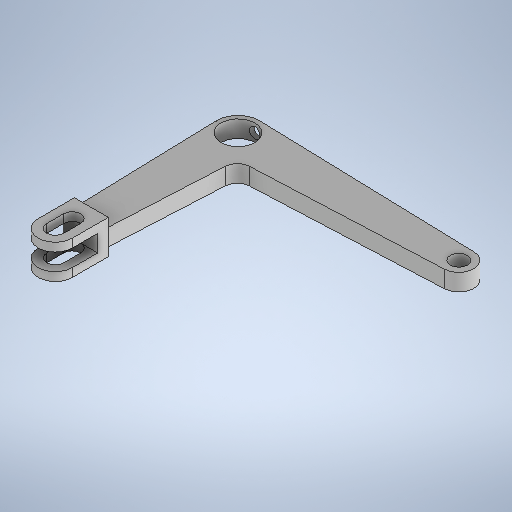
# Autodesk Inventor part: 10
Saved by Autodesk Inventor 2025.1 (Build 291241000, 241)
## iProperties
Created: 2024-09-12
Part Number: 10
Material: Generisch
Document SubType Name: Modeling
Designer: ffogue
Density: 1 g/cm^3
Appearance: Vorgabe
Author: ffogue
Autodesk Inventor part; units mm, degrees
ref_plane "YZ Plane" through (0, 0, 0) normal (1, 0, 0) x (0, 1, 0)
ref_plane "XZ Plane" through (0, 0, 0) normal (0, 1, 0) x (-1, 0, 0)
sketch "Sketch2" plane through (0, 0, 0) normal (0, 0, 1) x (1, 0, 0)
  line L0 (-4, 0) -> (4, 0)
  line L1 (4, 0) -> (4, -12.5)
  line L2 (4, -12.5) -> (-4, -12.5)
  line L3 (-4, -12.5) -> (-4, 0)
  point P0 (0, 0)
  point P1 (0, 0)
  dimension "d8" = 12.5
  dimension "d9" = 8
  constraints: 8 end point, 2 parallel, 1 coincident, 1 horizontal, 1 midpoint, 1 perpendicular
  measures "d8" distance between parallel lines of L2 L0
  measures "d9" distance of L0.start L0.end
extrude "Extrusion1" add sketch "Sketch2" along normal mid plane 8
fillet "Fillet1" radius 4 2 edges at (4, -12.5, 0) (-4, -12.5, 0)
sketch "Sketch4" plane through (0, 0, 4) normal (0, 0, 1) x (1, 0, 0)
  line L0 (0, -8.5) -> (0, -4.5) construction
  line L1 (2, -8.5) -> (2, -4.5)
  line L2 (-2, -4.5) -> (-2, -8.5)
  arc A0 (-2, -8.5) -> (2, -8.5) centre (0, -8.5) ccw
  arc A1 (2, -4.5) -> (-2, -4.5) centre (0, -4.5) ccw
  line L3 (4, 0) -> (-4, 0) projected
  point P0 (0, 0)
  point P1 (0, -6.5)
  point P2 (0, 0)
  dimension "d17" = 4
  dimension "d18" = 2
  constraints: 8 end point, 4 point on circle, 4 tangent, 2 centre point, 2 midpoint, 1 parallel, 1 vertical, 1 vertical alignment
  measures "d17" distance of L0.start L0.end
  measures "d18" radius of A0
extrude "Extrusion3" cut sketch "Sketch4" against normal blind 10
sketch "Sketch5" plane through (4, 0, 4) normal (1, 0, 0) x (0, 0, -1)
  line L0 (0, -8.5) -> (0, -8.5) projected
  line L1 (0, -8.5) -> (8, -8.5) projected
  line L2 (8, -8.5) -> (8, -8.5) projected
  line L3 (8, -8.5) -> (0, -8.5) projected
  line L4 (8, -12.5) -> (0, -12.5) projected
  line L5 (2, -2.5) -> (6, -2.5)
  line L6 (6, -2.5) -> (6, -12.5)
  line L7 (6, -12.5) -> (2, -12.5)
  line L8 (2, -12.5) -> (2, -2.5)
  line L9 (0, -8.5) -> (0, 0) projected
  point P0 (4, 0)
  dimension "d22" = 4
  dimension "d23" = 10
  dimension "d24" = 2
  constraints: 8 end point, 2 parallel, 1 horizontal, 1 perpendicular, 1 point on line
  measures "d22" distance of L5.start L5.end
  measures "d23" distance between parallel lines of L4 L5
  measures "d24" distance between parallel lines of L9 L8
extrude "Extrusion4" cut sketch "Sketch5" against normal up to surface (8 mm away)
ref_plane "Work Plane1" through (0, 0, 0) normal (0, 0, 1) x (1, 0, 0)
sketch "Sketch6" plane through (0, 0, 0) normal (0, 0, 1) x (1, 0, 0)
  line L0 (-4, 0) -> (4, 0) projected
  line L1 (-4, 0) -> (-4.9979, 34.3548)
  arc A0 (0, 39.5) -> (-4.9979, 34.3548) centre (0, 34.5) ccw
  line L2 (0, 39.5) -> (52.1008, 37.9985)
  arc A1 (52.1585, 31.0036) -> (52.1008, 37.9985) centre (52, 34.5) ccw
  line L3 (52.1585, 31.0036) -> (8.2033, 29.0116)
  line L4 (5.343, 26.1684) -> (4, 0)
  arc A2 (0, -2.5) -> (-2, -4.5) centre (0, -4.5) ccw projected
  arc A3 (2, -4.5) -> (0, -2.5) centre (0, -4.5) ccw projected
  arc A4 (8.2033, 29.0116) -> (5.343, 26.1684) centre (8.3391, 26.0147) ccw
  point P0 (0, 0)
  point P1 (0, 0)
  dimension "d28" = 5
  dimension "d29" = 39
  dimension "d30" = 52
  dimension "d31" = 3
  dimension "d32" = 3.5
  constraints: 8 end point, 6 point on circle, 5 tangent, 3 centre point, 2 vertical alignment, 1 horizontal alignment, 1 midpoint
  measures "d28" radius of A0
  measures "d29" distance of A2.centre A0.centre
  measures "d30" distance of A1.centre A0.centre
  measures "d31" radius of A4
  measures "d32" radius of A1
extrude "Extrusion5" add sketch "Sketch6" along normal mid plane 4
sketch "Sketch7" plane through (0, 0, 2) normal (0, 0, 1) x (1, 0, 0)
  arc A0 (52.1585, 31.0036) -> (52.1008, 37.9985) centre (52, 34.5) ccw projected
  point P0 (0, 0)
  constraints: 1 coincident
hole "Hole1" at (52, 34.5, 2) direction (0, 0, -1) diameter 4 depth 4
sketch "Sketch8" plane through (0, 0, 2) normal (0, 0, 1) x (1, 0, 0)
  arc A0 (0, 39.5) -> (-4.9979, 34.3548) centre (0, 34.5) ccw projected
  point P0 (0, 0)
  constraints: 1 coincident
hole "Hole2" at (0, 34.5, 2) direction (0, 0, -1) diameter 8 depth 4
sketch "Sketch9" plane through (0, 39.5, 2) normal (0.0288, 0.9996, 0) x (0.9996, -0.0288, 0)
  line L0 (-4.8476, 0) -> (-4.8476, 4) projected
  line L1 (4.144, 0) -> (-3.856, 0) projected
  point P0 (1.1378, 2)
  point P1 (0.144, 2)
  point P2 (-4.8476, 2)
  point P3 (0.144, 0)
  constraints: 2 midpoint, 1 horizontal alignment, 1 vertical alignment
hole "Hole3" at (0.144, 39.4959, 0) direction (-0.0288, -0.9996, 0) diameter 2.5 depth 12
sketch "Sketch10" plane through (0, 0, -4) normal (0, 0, 1) x (1, 0, 0)
  circle A0 centre (0, -6.592) radius 2
  line L0 (4, 0) -> (-4, 0) projected
  line L1 (-2, -4.5) -> (-2, -8.5) projected
  arc A1 (-2, -8.5) -> (2, -8.5) centre (0, -8.5) ccw projected
  point P0 (0, 0)
  point P1 (0, 0)
  point P2 (-2, -6.5)
  point P3 (0, -10.5)
  dimension "d57" = 4
  dimension "d59" = 3.908
  constraints: 2 midpoint, 1 centre point, 1 point on circle, 1 vertical alignment
  measures "d57" diameter of A0
  measures "d59" distance of point (0, -10.5) A0.centre
body "Solid1"
